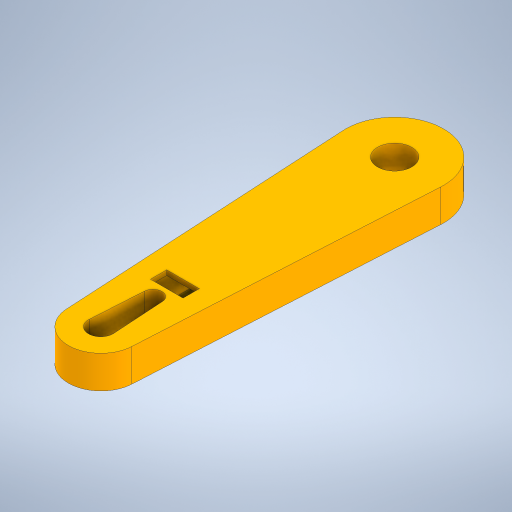
# Autodesk Inventor part: Brazo
Saved by Autodesk Inventor 2024 (Build 280153000, 153)
## iProperties
Created: 2024-04-28
Part Number: Brazo
Material: Generic
Document SubType Name: Modeling
Designer: samue
Density: 1 g/cm^3
Appearance: Default
Author: samue
## iProperties of the stored document Brazo_3DPrint.ipt
Created: 2024-04-28
Part Number: Brazo_3DPrint
Material: Generic
Document SubType Name: Modeling
Designer: samue
Density: 1 g/cm^3
Appearance: Default
Author: samue
Autodesk Inventor part; units mm, degrees
ref_plane "YZ Plane" through (0, 0, 0) normal (1, 0, 0) x (0, 1, 0)
ref_plane "XZ Plane" through (0, 0, 0) normal (0, 1, 0) x (-1, 0, 0)
sketch "Sketch1" plane through (0, 0, 0) normal (0, 1, 0) x (-1, 0, 0)
  circle A0 centre (-0.0087, 99.7911) radius 10
  circle A1 centre (-0.0022, 9.7911) radius 15
  line L0 (9.9759, 100.3474) -> (14.9746, 10.6255)
  line L1 (-9.9933, 100.346) -> (-14.9791, 10.6234)
  point P0 (0, 0)
  dimension "d0" = 20
  dimension "d1" = 30
  dimension "d2" = 90
  constraints: 4 end point, 4 point on circle, 4 tangent, 2 centre point
  measures "d0" diameter of A0
  measures "d1" diameter of A1
  measures "d2" distance of A1.centre A0.centre
extrude "Extrusion1" add sketch "Sketch1" against normal blind 10
sketch "Sketch2" plane through (0, 0, 0) normal (0, 1, 0) x (1, 0, 0)
  circle A0 centre (0, -99.8683) radius 3.75
  circle A1 centre (0, -83.8683) radius 2.75
  line L0 (2.7446, -83.6964) -> (3.7427, -99.6339)
  line L1 (-3.7427, -99.6339) -> (-2.7446, -83.6964)
  point P0 (0, 0)
  dimension "d7" = 7.5
  dimension "d8" = 5.5
  dimension "d9" = 16
  constraints: 4 end point, 4 point on circle, 4 tangent, 2 centre point
  measures "d7" diameter of A0
  measures "d8" diameter of A1
  measures "d9" distance of A0.centre A1.centre
extrude "Extrusion2" cut sketch "Sketch2" against normal blind 8.5
sketch "Sketch3" plane through (0, -8.5, 0) normal (0, 1, 0) x (1, 0, 0)
  arc A0 (-3.7427, -99.6339) -> (3.7427, -99.6339) centre (0, -99.8683) ccw projected
  circle A1 centre (0, -99.8683) radius 3.65
  point P0 (0, 0)
  dimension "d12" = 7.3
  constraints: 1 centre point, 1 coincident
  measures "d12" diameter of A1
extrude "Extrusion3" cut sketch "Sketch3" against normal blind 8.5
sketch "Sketch4" plane through (0, 0, 0) normal (0, 1, 0) x (1, 0, 0)
  arc A0 (14.9791, -10.6234) -> (-14.9746, -10.6255) centre (0.0022, -9.7911) ccw projected
  circle A1 centre (0.0022, -9.7911) radius 5.25
  point P0 (0, 0)
  dimension "d15" = 10.5
  constraints: 1 centre point, 1 coincident
  measures "d15" diameter of A1
extrude "Extrusion4" cut sketch "Sketch4" against normal blind 11
sketch "Sketch6" plane through (0, 0, 0) normal (0, 0, 1) x (1, 0, 0)
  line L0 (-10.7414, -1.5061) -> (11.4058, -1.5061)
  line L1 (11.4058, -1.5061) -> (11.4058, -8.375)
  line L2 (11.4058, -8.375) -> (-10.7414, -8.375)
  line L3 (-10.7414, -8.375) -> (-10.7414, -1.5061)
  point P0 (0, 0)
  constraints: 8 end point, 2 parallel, 1 horizontal, 1 perpendicular
extrude "Extrusion6" add sketch "Sketch6" along normal blind 1
ref_plane "Work Plane3" through (0, 0, 79.75) normal (0, 0, -1) x (-1, 0, 0)
sketch "Sketch7" plane through (0, 0, 79.75) normal (0, 0, -1) x (-1, 0, 0)
  line L0 (5.25, -1.5083) -> (-5.25, -1.5083)
  line L1 (-5.25, -1.5083) -> (-5.25, -8.8083)
  line L2 (-5.25, -8.8083) -> (5.25, -8.8083)
  line L3 (5.25, -8.8083) -> (5.25, -1.5083)
  line L4 (5.25, -1.5083) -> (-5.25, -8.8083) construction
  line L5 (-5.25, -1.5083) -> (5.25, -8.8083) construction
  point P0 (0, 0)
  point P1 (0, -5.1583)
  dimension "d23" = 10.5
  dimension "d24" = 7.3
  constraints: 12 end point, 2 midpoint, 2 parallel, 1 horizontal, 1 perpendicular
  measures "d23" distance of L2.end L1.end
  measures "d24" distance of L1.end L0.end
extrude "Extrusion7" cut sketch "Sketch7" along normal blind 62.25
sketch "Sketch8" plane through (0, 0, 0) normal (0, 1, 0) x (1, 0, 0)
  line L0 (-5, -79.6503) -> (5, -79.6503)
  line L1 (5, -79.6503) -> (5, -74.6503)
  line L2 (5, -74.6503) -> (-5, -74.6503)
  line L3 (-5, -74.6503) -> (-5, -79.6503)
  line L4 (-5, -79.6503) -> (5, -74.6503) construction
  line L5 (5, -79.6503) -> (-5, -74.6503) construction
  point P0 (0, 0)
  point P1 (0, -77.1503)
  dimension "d27" = 10
  dimension "d28" = 5
  constraints: 12 end point, 2 midpoint, 2 parallel, 1 horizontal, 1 perpendicular
  measures "d27" distance of L2.end L1.end
  measures "d28" distance of L1.end L0.end
extrude "Extrusion8" cut sketch "Sketch8" against normal blind 8.5
sketch "Sketch9" plane through (-14.9746, -10, 10.6255) normal (-0.9985, 0, 0.0556) x (0.0556, 0, 0.9985)
  line L0 (16.1756, 2.6337) -> (6.1756, 2.6337)
  line L1 (6.1756, 2.6337) -> (6.1756, 7.6337)
  line L2 (6.1756, 7.6337) -> (16.1756, 7.6337)
  line L3 (16.1756, 7.6337) -> (16.1756, 2.6337)
  line L4 (16.1756, 2.6337) -> (6.1756, 7.6337) construction
  line L5 (6.1756, 2.6337) -> (16.1756, 7.6337) construction
  point P0 (-9.7761, 10)
  point P1 (11.1756, 5.1337)
  dimension "d31" = 10
  dimension "d32" = 5
  constraints: 12 end point, 2 midpoint, 2 parallel, 1 horizontal, 1 perpendicular
  measures "d31" distance of L1.end L2.end
  measures "d32" distance of L0.end L1.end
extrude "Extrusion9" cut sketch "Sketch9" against normal blind 20.5
body "Solid1"
